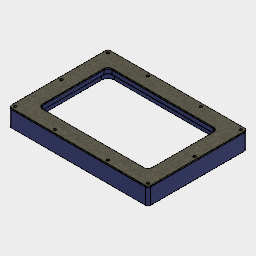
filter_inlet (Autodesk Fusion 360 design; units mm, degrees)
Autodesk Fusion 360 part; units mm, degrees
sketch "the main event" plane through (0, 0, 0) normal (0, 1, 0) x (1, 0, 0)
  line L0 (0, 0) -> (158, 0)
  line L1 (158, 0) -> (158, -108)
  line L2 (158, -108) -> (0, -108)
  line L3 (0, -108) -> (0, 0)
  circle A0 centre (46, 4) radius 2.75
  line L4 (-8, 8) -> (166, 8)
  line L5 (166, 8) -> (166, -116)
  line L6 (166, -116) -> (-8, -116)
  line L7 (-8, -116) -> (-8, 8)
  line L8 (147.5, -97.5) -> (10.5, -97.5)
  line L9 (10.5, -97.5) -> (10.5, -10.5)
  line L10 (10.5, -10.5) -> (147.5, -10.5)
  line L11 (147.5, -10.5) -> (147.5, -97.5)
  line L12 (-4, 4) -> (162, 4) construction
  line L13 (162, 4) -> (162, -112) construction
  line L14 (162, -112) -> (-4, -112) construction
  line L15 (-4, -112) -> (-4, 4) construction
  dimension "d1" = 158
  dimension "d2" = 108
  dimension "d3" = 8
  dimension "d4" = 10.5
  dimension "d18" = 50
  dimension "d19" = 50
  dimension "d36" = 4
  dimension "d37" = 5.5
  constraint horizontal L0
  constraint vertical L1
  constraint horizontal L2
  constraint vertical L3
  constraint coincident L0.start L3.end
  constraint coincident L14
  constraint midpoint L0.start L15
  constraint midpoint L0.start L13
  constraint coincident L0.start L12
  constraint vertical L0.start
  measures "d18" distance of L0.start L13
  measures "d19" distance of L0.start L15
  measures "d36" distance of L2 L14
  measures "d37" diameter of A0
extrude "Extrude1" add sketch "the main event" along normal blind 5 contours L0 L1 L2 L3 | A0 | L4 L5 L6 L7 makes body 1
extrude "Extrude2" add sketch "the main event" against normal blind 15 contours A0 | L4 L5 L6 L7 bodies 1
fillet "Fillet1" radius 3 4 edges at (-8, -5, 116) (-8, -5, -8) (166, -5, -8) (166, -5, 116) on bodies 1
fillet "Fillet1" radius 5 4 edges at (10.5, 2.5, 10.5) (10.5, 2.5, 97.5) (147.5, 2.5, 10.5) (147.5, 2.5, 97.5) on bodies 1
fillet "Fillet1" radius 8 4 edges at (0, -7.5, 108) (0, -7.5, 0) (158, -7.5, 0) (158, -7.5, 108) on bodies 1
sketch "projected for countersink hole" plane through (0, -15, 0) normal (0, -1, 0) x (1, 0, 0)
  line L0 (8, 108) -> (150, 108)
  line L1 (158, 100) -> (158, 8)
  line L2 (150, 0) -> (8, 0)
  line L3 (0, 8) -> (0, 100)
  arc A0 (166, 113) -> (163, 116) centre (163, 113) ccw
  line L4 (163, 116) -> (-5, 116)
  arc A1 (-5, 116) -> (-8, 113) centre (-5, 113) ccw
  line L5 (-8, 113) -> (-8, -5)
  arc A2 (-8, -5) -> (-5, -8) centre (-5, -5) ccw
  line L6 (-5, -8) -> (163, -8)
  arc A3 (163, -8) -> (166, -5) centre (163, -5) ccw
  line L7 (166, -5) -> (166, 113)
  arc A4 (158, 100) -> (150, 108) centre (150, 100) ccw
  arc A5 (150, 0) -> (158, 8) centre (150, 8) ccw
  arc A6 (0, 8) -> (8, 0) centre (8, 8) ccw
  arc A7 (8, 108) -> (0, 100) centre (8, 100) ccw
hole "Hole1" at (112, -15, -4) at (162, -15, -4) at (162, -15, 112) at (112, -15, 112) at (46, -15, 112) at (-4, -15, 112) at (-4, -15, -4) at (46, -15, -4) at (-4, -15, 54) at (162, -15, 54) direction (0, 1, 0) diameter 3.2 end through all bodies 1
sketch "projected for gasket_dxf" plane through (0, 0, 0) normal (0, 1, 0) x (1, 0, 0)
  circle A0 centre (-4, 4) radius 1.6
  circle A1 centre (46, -112) radius 1.6
  circle A2 centre (162, -112) radius 1.6
  circle A3 centre (112, 4) radius 1.6
  circle A4 centre (162, 4) radius 1.6
  circle A5 centre (112, -112) radius 1.6
  circle A6 centre (-4, -112) radius 1.6
  circle A7 centre (46, 4) radius 1.6
  arc A8 (163, -116) -> (166, -113) centre (163, -113) ccw
  line L0 (166, -113) -> (166, 5)
  arc A9 (166, 5) -> (163, 8) centre (163, 5) ccw
  line L1 (163, 8) -> (-5, 8)
  arc A10 (-5, 8) -> (-8, 5) centre (-5, 5) ccw
  line L2 (-8, 5) -> (-8, -113)
  arc A11 (-8, -113) -> (-5, -116) centre (-5, -113) ccw
  line L3 (-5, -116) -> (163, -116)
  line L4 (15.5, -10.5) -> (142.5, -10.5)
  arc A12 (147.5, -15.5) -> (142.5, -10.5) centre (142.5, -15.5) ccw
  line L5 (147.5, -15.5) -> (147.5, -92.5)
  arc A13 (142.5, -97.5) -> (147.5, -92.5) centre (142.5, -92.5) ccw
  line L6 (142.5, -97.5) -> (15.5, -97.5)
  arc A14 (10.5, -92.5) -> (15.5, -97.5) centre (15.5, -92.5) ccw
  line L7 (10.5, -92.5) -> (10.5, -15.5)
  arc A15 (15.5, -10.5) -> (10.5, -15.5) centre (15.5, -15.5) ccw
  circle A16 centre (-4, -54) radius 1.6
  circle A17 centre (162, -54) radius 1.6
extrude "Extrude3" add 1 faces at (157.7, 5, 86.1667) along direction (0, 1, 0) blind 1.6 separate body on bodies 1 makes body 2
ref_plane "WorkPlane3" through (79, -5, 54) normal (0, -1, 0) x (0, 0, -1)
ref_plane "WorkPlane4" through (79, 3, 54) normal (0, -1, 0) x (0, 0, -1)
sketch "middle_dxf" plane through (77, -5, 52) normal (0, -1, 0) x (1, 0, 0)
  circle A0 centre (-81, 2) radius 1.6
  circle A1 centre (-81, -56) radius 1.6
  circle A2 centre (-31, 60) radius 1.6
  circle A3 centre (85, 60) radius 1.6
  circle A4 centre (35, -56) radius 1.6
  circle A5 centre (85, -56) radius 1.6
  circle A6 centre (35, 60) radius 1.6
  circle A7 centre (-81, 60) radius 1.6
  circle A8 centre (-31, -56) radius 1.6
  circle A9 centre (85, 2) radius 1.6
  arc A10 (73, 56) -> (81, 48) centre (73, 48) cw
  line L0 (81, 48) -> (81, -44)
  arc A11 (81, -44) -> (73, -52) centre (73, -44) cw
  line L1 (73, -52) -> (-69, -52)
  arc A12 (-69, -52) -> (-77, -44) centre (-69, -44) cw
  line L2 (-77, -44) -> (-77, 48)
  arc A13 (-77, 48) -> (-69, 56) centre (-69, 48) cw
  line L3 (-69, 56) -> (73, 56)
  arc A14 (89, 61) -> (86, 64) centre (86, 61) ccw
  line L4 (86, 64) -> (-82, 64)
  arc A15 (-82, 64) -> (-85, 61) centre (-82, 61) ccw
  line L5 (-85, 61) -> (-85, -57)
  arc A16 (-85, -57) -> (-82, -60) centre (-82, -57) ccw
  line L6 (-82, -60) -> (86, -60)
  arc A17 (86, -60) -> (89, -57) centre (86, -57) ccw
  line L7 (89, -57) -> (89, 61)
sketch "bottom and gasket dxf" plane through (77, 3, 54) normal (0, -1, 0) x (1, 0, 0)
  circle A0 centre (-81, 0) radius 1.6
  circle A1 centre (-81, -58) radius 1.6
  circle A2 centre (-31, 58) radius 1.6
  circle A3 centre (85, 58) radius 1.6
  circle A4 centre (35, -58) radius 1.6
  circle A5 centre (85, -58) radius 1.6
  circle A6 centre (35, 58) radius 1.6
  circle A7 centre (-81, 58) radius 1.6
  circle A8 centre (-31, -58) radius 1.6
  circle A9 centre (85, 0) radius 1.6
  arc A10 (70.5, 38.5) -> (65.5, 43.5) centre (65.5, 38.5) ccw
  line L0 (65.5, 43.5) -> (-61.5, 43.5)
  arc A11 (65.5, -43.5) -> (70.5, -38.5) centre (65.5, -38.5) ccw
  line L1 (70.5, -38.5) -> (70.5, 38.5)
  arc A12 (-61.5, 43.5) -> (-66.5, 38.5) centre (-61.5, 38.5) ccw
  line L2 (-66.5, 38.5) -> (-66.5, -38.5)
  arc A13 (-66.5, -38.5) -> (-61.5, -43.5) centre (-61.5, -38.5) ccw
  line L3 (-61.5, -43.5) -> (65.5, -43.5)
  arc A14 (89, 59) -> (86, 62) centre (86, 59) ccw
  line L4 (89, 59) -> (89, -59)
  arc A15 (86, -62) -> (89, -59) centre (86, -59) ccw
  line L5 (86, -62) -> (-82, -62)
  arc A16 (-85, -59) -> (-82, -62) centre (-82, -59) ccw
  line L6 (-85, -59) -> (-85, 59)
  arc A17 (-82, 62) -> (-85, 59) centre (-82, 59) ccw
  line L7 (-82, 62) -> (86, 62)
sketch "clamp" plane through (0, -15, 0) normal (0, -1, 0) x (1, 0, 0)
  circle A0 centre (-4.6254, -4.6254) radius 2.85
  circle A1 centre (45.3746, 108.6254) radius 2.85
  circle A2 centre (158.6254, 108.6254) radius 2.85
  circle A3 centre (108.6254, -4.6254) radius 2.85
  circle A4 centre (158.6254, -4.6254) radius 2.85
  circle A5 centre (108.6254, 108.6254) radius 2.85
  circle A6 centre (-4.6254, 108.6254) radius 2.85
  circle A7 centre (45.3746, -4.6254) radius 2.85
  line L0 (2, 104) -> (152, 104)
  line L1 (154, 102) -> (154, 2)
  line L2 (152, 0) -> (2, 0)
  line L3 (0, 2) -> (0, 102)
  arc A8 (164, 111) -> (161, 114) centre (161, 111) ccw
  line L4 (161, 114) -> (-7, 114)
  arc A9 (-7, 114) -> (-10, 111) centre (-7, 111) ccw
  line L5 (-10, 111) -> (-10, -7)
  arc A10 (-10, -7) -> (-7, -10) centre (-7, -7) ccw
  line L6 (-7, -10) -> (161, -10)
  arc A11 (161, -10) -> (164, -7) centre (161, -7) ccw
  line L7 (164, -7) -> (164, 111)
  line L8 (154.1254, 52) -> (154.1254, 81.6606)
  line L9 (162.5225, 49.75) -> (177.3528, 75.4368)
  arc A12 (177.3528, 75.4368) -> (154.1254, 81.6606) centre (158.6254, 52) ccw
  arc A13 (154.1254, 52) -> (162.5225, 49.75) centre (158.6254, 52) ccw
  circle A14 centre (-4.6254, 52) radius 2.85
  circle A15 centre (158.6254, 52) radius 2.85
  arc A16 (154, 102) -> (152, 104) centre (152, 102) ccw
  arc A17 (152, 0) -> (154, 2) centre (152, 2) ccw
  arc A18 (0, 2) -> (2, 0) centre (2, 2) ccw
  arc A19 (2, 104) -> (0, 102) centre (2, 102) ccw
  dimension "d25" = 9
  dimension "d26" = 30
  dimension "d27" = 30
  constraint parallel L1 L8
  constraint tangent L9 A13
  constraint tangent L8 A13
  measures "d25" diameter of A13
  measures "d26" radius of A12
  measures "d27" angle of L8 L9
extrude "Extrude4" [suppressed]
fillet "Fillet2" [suppressed]
ref_plane "WorkPlane1" through (77, -5, 52) normal (0, -1, 0) x (0, 0, -1)
ref_plane "WorkPlane2" through (77, 4, 52) normal (0, -1, 0) x (0, 0, -1)
sketch "laser_cut_filter_bulkhead_bot" plane through (75, 4, 50) normal (0, -1, 0) x (1, 0, 0)
  circle A0 centre (83.6254, 2) radius 1.6
  circle A1 centre (-79.6254, 2) radius 1.6
  circle A2 centre (-79.6254, -54.6254) radius 1.6
  circle A3 centre (-29.6254, 58.6254) radius 1.6
  circle A4 centre (83.6254, 58.6254) radius 1.6
  circle A5 centre (33.6254, -54.6254) radius 1.6
  circle A6 centre (83.6254, -54.6254) radius 1.6
  circle A7 centre (33.6254, 58.6254) radius 1.6
  circle A8 centre (-79.6254, 58.6254) radius 1.6
  circle A9 centre (-29.6254, -54.6254) radius 1.6
  arc A10 (72.5, -38.5) -> (67.5, -43.5) centre (67.5, -38.5) cw
  line L0 (67.5, -43.5) -> (-63.5, -43.5)
  arc A11 (-63.5, -43.5) -> (-68.5, -38.5) centre (-63.5, -38.5) cw
  line L1 (-68.5, -38.5) -> (-68.5, 42.5)
  arc A12 (-68.5, 42.5) -> (-63.5, 47.5) centre (-63.5, 42.5) cw
  line L2 (-63.5, 47.5) -> (67.5, 47.5)
  arc A13 (67.5, 47.5) -> (72.5, 42.5) centre (67.5, 42.5) cw
  line L3 (72.5, 42.5) -> (72.5, -38.5)
  arc A14 (89, 59) -> (84, 64) centre (84, 59) ccw
  line L4 (84, 64) -> (-80, 64)
  arc A15 (-80, 64) -> (-85, 59) centre (-80, 59) ccw
  line L5 (-85, 59) -> (-85, -55)
  arc A16 (-85, -55) -> (-80, -60) centre (-80, -55) ccw
  line L6 (-80, -60) -> (84, -60)
  arc A17 (84, -60) -> (89, -55) centre (84, -55) ccw
  line L7 (89, -55) -> (89, 59)
sketch "laser_cut_filter_bulkhead_top" plane through (75, -5, 50) normal (0, -1, 0) x (1, 0, 0)
  circle A0 centre (83.6254, 2) radius 1.6
  circle A1 centre (-79.6254, 2) radius 1.6
  circle A2 centre (-79.6254, -54.6254) radius 1.6
  circle A3 centre (-29.6254, 58.6254) radius 1.6
  circle A4 centre (83.6254, 58.6254) radius 1.6
  circle A5 centre (33.6254, -54.6254) radius 1.6
  circle A6 centre (83.6254, -54.6254) radius 1.6
  circle A7 centre (33.6254, 58.6254) radius 1.6
  circle A8 centre (-79.6254, 58.6254) radius 1.6
  circle A9 centre (-29.6254, -54.6254) radius 1.6
  arc A10 (89, 59) -> (84, 64) centre (84, 59) ccw
  line L0 (84, 64) -> (-80, 64)
  arc A11 (-80, 64) -> (-85, 59) centre (-80, 59) ccw
  line L1 (-85, 59) -> (-85, -55)
  arc A12 (-85, -55) -> (-80, -60) centre (-80, -55) ccw
  line L2 (-80, -60) -> (84, -60)
  arc A13 (84, -60) -> (89, -55) centre (84, -55) ccw
  line L3 (89, -55) -> (89, 59)
  line L4 (-75, -50) -> (-75, 54)
  line L5 (-75, 54) -> (79, 54)
  line L6 (79, 54) -> (79, -50)
  line L7 (79, -50) -> (-75, -50)
